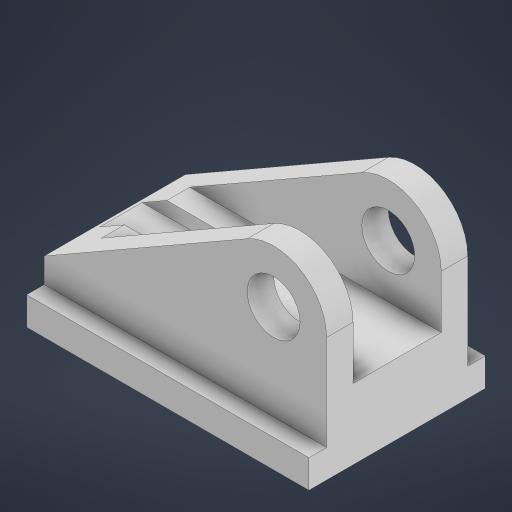
# Autodesk Inventor part: Część7
Saved by Autodesk Inventor 2023 (Build 270158000, 158)
## iProperties
Created: 2023-05-07
Part Number: Część7
Material: Ogólny
Document SubType Name: Modeling
Designer: Adam
Density: 1 g/cm^3
Appearance: Domyślna
Author: Adam
Autodesk Inventor part; units mm, degrees
ref_plane "YZ Plane" through (0, 0, 0) normal (1, 0, 0) x (0, 1, 0)
ref_plane "XZ Plane" through (0, 0, 0) normal (0, 1, 0) x (-1, 0, 0)
ref_plane "XY Plane" through (0, 0, 0) normal (0, 0, 1) x (1, 0, 0)
sketch "Szkic1" plane through (0, 0, 0) normal (0, 1, 0) x (-1, 0, 0)
  line L0 (40, -25) -> (-40, -25)
  line L1 (-40, -25) -> (-40, 25)
  line L2 (-40, 25) -> (40, 25)
  line L3 (40, 25) -> (40, -25)
  point P0 (0, 0)
  dimension "d0" = 80
  dimension "d1" = 50
  constraints: 8 end point, 2 parallel, 1 horizontal, 1 perpendicular
  measures "d0" distance of L1.end L2.end
  measures "d1" distance of L0.end L1.end
extrude "Wyciągnięcie proste1" add sketch "Szkic1" along normal blind 8
sketch "Szkic2" plane through (0, 8, 0) normal (0, 1, 0) x (1, 0, 0)
  line L0 (40, -25) -> (40, 25) projected
  line L1 (-40, -20) -> (40, -20)
  line L2 (40, -20) -> (40, 20)
  line L3 (40, 20) -> (-40, 20)
  line L4 (-40, 20) -> (-40, -20)
  line L5 (-40, -20) -> (40, 20) construction
  line L6 (40, -20) -> (-40, 20) construction
  point P0 (0, 0)
  dimension "d4" = 40
  constraints: 12 end point, 2 midpoint, 2 parallel, 1 horizontal, 1 perpendicular, 1 point on line
  measures "d4" distance of L2.end L1.end
extrude "Wyciągnięcie proste2" add sketch "Szkic2" along normal blind 42
sketch "Szkic3" plane through (-40, 8, 20) normal (0, 0, 1) x (1, 0, 0)
  line L0 (0, 0) -> (0, 42) projected
  line L1 (0, 0) -> (0, 7)
  circle A0 centre (65, 27) radius 15
  line L2 (80, 0) -> (80, 42) projected
  line L3 (0, 42) -> (80, 42) projected
  line L4 (0, 7) -> (57.5352, 40.0106)
  point P0 (40, -8)
  point P1 (65, 42)
  point P2 (80, 27)
  dimension "d8" = 30
  dimension "d7" = 7
  constraints: 4 end point, 1 horizontal, 1 point on line, 1 vertical, 4 other
  measures "d7" distance of L0.start L1.end
extrude "Wyciągnięcie proste3" cut sketch "Szkic3" against normal through all contours L0 L3 A0 L4 | L3 L2 A0
sketch "Szkic4" plane through (40, 0, 25) normal (1, 0, 0) x (0, 0, -1)
  line L0 (12.5, 20) -> (37.5, 20)
  line L1 (37.5, 20) -> (37.5, 50)
  line L2 (37.5, 50) -> (12.5, 50)
  line L3 (12.5, 50) -> (12.5, 20)
  line L4 (12.5, 20) -> (37.5, 50) construction
  line L5 (37.5, 20) -> (12.5, 50) construction
  line L6 (0, 0) -> (50, 0) projected
  point P0 (25, 0)
  point P1 (25, 35)
  dimension "d11" = 25
  dimension "d12" = 30
  dimension "d13" = 20
  constraints: 12 end point, 2 midpoint, 2 parallel, 1 horizontal, 1 perpendicular
  measures "d11" distance of L2.end L1.end
  measures "d12" distance of L1.end L0.end
  measures "d13" distance between parallel lines of L0 L6
sketch "Szkic5" plane through (-40, 8, 20) normal (0, 0, 1) x (1, 0, 0)
  arc A0 (80, 27) -> (57.5352, 40.0106) centre (65, 27) ccw projected
  point P0 (40, -8)
  constraints: 1 coincident
extrude "Wyciągnięcie proste4" cut sketch "Szkic4" against normal through all
sketch "Szkic6" plane through (40, 20, 12.5) normal (0, 1, 0) x (1, 0, 0)
  line L0 (-55, 18.5) -> (-80, 18.5)
  line L1 (-80, 18.5) -> (-80, 6.5)
  line L2 (-80, 6.5) -> (-55, 6.5)
  line L3 (-55, 6.5) -> (-55, 18.5)
  line L4 (-55, 18.5) -> (-80, 6.5) construction
  line L5 (-80, 18.5) -> (-55, 6.5) construction
  line L6 (0, 25) -> (0, 0) projected
  point P0 (-40, 12.5)
  point P1 (-67.5, 12.5)
  point P2 (-55, 12.5)
  dimension "d16" = 25
  dimension "d17" = 55
  dimension "d18" = 12
  constraints: 12 end point, 3 midpoint, 2 parallel, 1 horizontal, 1 perpendicular
  measures "d16" distance of L2.end L1.end
  measures "d17" distance from line of point (-55, 12.5) L6
  measures "d18" distance of L2.end L0.start
extrude "Wyciągnięcie proste5" cut sketch "Szkic6" against normal blind 4
hole "Otwór1" at (25, 35, 20) direction (0, 0, -1) diameter 15 end through all
